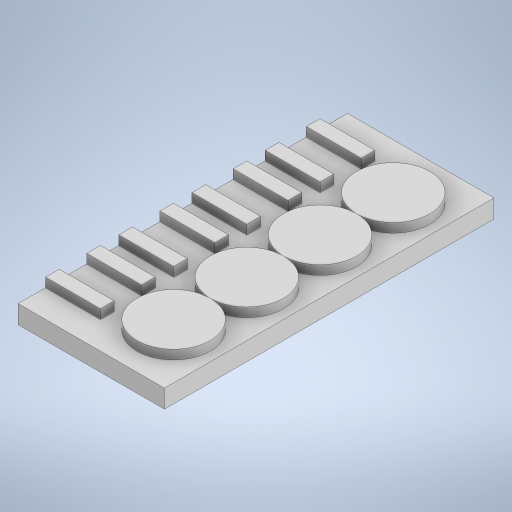
# Autodesk Inventor part: Zamysl na rekina
Saved by Autodesk Inventor 2024 (Build 280153000, 153)
## iProperties
Created: 2023-10-15
Part Number: Zamysl na rekina
Material: Generic
Document SubType Name: Modeling
Designer: Piter
Density: 1 g/cm^3
Appearance: Default
Author: Piter
Autodesk Inventor part; units mm, degrees
ref_plane "YZ Plane" through (0, 0, 0) normal (1, 0, 0) x (0, 1, 0)
ref_plane "XZ Plane" through (0, 0, 0) normal (0, 1, 0) x (-1, 0, 0)
ref_plane "XY Plane" through (0, 0, 0) normal (0, 0, 1) x (1, 0, 0)
sketch "Sketch1" plane through (0, 0, 0) normal (0, 1, 0) x (-1, 0, 0)
  line L0 (71.2912, 117.5402) -> (-8.7088, 117.5402)
  line L1 (-8.7088, 117.5402) -> (-8.7088, -62.4598)
  line L2 (-8.7088, -62.4598) -> (71.2912, -62.4598)
  line L3 (71.2912, -62.4598) -> (71.2912, 117.5402)
  point P0 (0, 0)
  dimension "d0" = 80
  dimension "d1" = 180
  constraints: 8 end point, 2 parallel, 1 horizontal, 1 perpendicular
  measures "d0" distance of L2.end L1.end
  measures "d1" distance of L1.end L0.end
extrude "Extrusion1" add sketch "Sketch1" along normal blind 10
sketch "Sketch2" plane through (0, 10, 0) normal (0, 1, 0) x (1, 0, 0)
  line L0 (8.7088, -117.5402) -> (8.7088, 62.4598) projected
  line L1 (8.7088, 62.4598) -> (-71.2912, 62.4598) projected
  line L2 (8.7088, -117.5402) -> (-16.2912, -117.5402)
  line L3 (-16.2912, 62.4598) -> (8.7088, 62.4598)
  line L4 (8.7088, 62.4598) -> (8.7088, -117.5402)
  line L5 (-16.2912, -117.5402) -> (-16.2912, -87.5402)
  circle A0 centre (-16.2912, -87.5402) radius 20
  circle A1 centre (-16.2912, -47.5402) radius 20
  circle A2 centre (-16.2912, -7.5402) radius 20
  circle A3 centre (-16.2912, 32.4598) radius 20
  line L6 (-16.2912, -87.5402) -> (-70.5888, -87.5402)
  line L7 (-71.2912, 62.4598) -> (-71.2912, -117.5402) projected
  line L8 (-41.2912, -95.0402) -> (-71.2912, -95.0402)
  line L9 (-71.2912, -95.0402) -> (-71.2912, -80.0402)
  line L10 (-71.2912, -80.0402) -> (-41.2912, -80.0402)
  line L11 (-41.2912, -80.0402) -> (-41.2912, -95.0402)
  line L12 (-41.2912, -95.0402) -> (-71.2912, -80.0402) construction
  line L13 (-71.2912, -95.0402) -> (-41.2912, -80.0402) construction
  line L14 (-71.2912, -95.0402) -> (-41.2912, -95.0402)
  line L15 (-41.2912, -95.0402) -> (-41.2912, -102.5402)
  line L16 (-41.2912, -102.5402) -> (-71.2912, -102.5402)
  line L17 (-71.2912, -102.5402) -> (-71.2912, -95.0402)
  line L18 (-71.2912, -80.0402) -> (-41.2912, -80.0402)
  line L19 (-41.2912, -80.0402) -> (-41.2912, -72.5402)
  line L20 (-41.2912, -72.5402) -> (-71.2912, -72.5402)
  line L21 (-71.2912, -72.5402) -> (-71.2912, -80.0402)
  line L22 (-41.2912, -40.0402) -> (-41.2912, -32.5402)
  line L23 (-41.2912, -32.5402) -> (-71.2912, -32.5402)
  line L24 (-71.2912, -32.5402) -> (-71.2912, -40.0402)
  line L25 (-71.2912, -40.0402) -> (-41.2912, -40.0402)
  line L26 (-71.2912, -40.0402) -> (-41.2912, -40.0402)
  line L27 (-41.2912, -40.0402) -> (-41.2912, -55.0402)
  line L28 (-41.2912, -55.0402) -> (-41.2912, -62.5402)
  line L29 (-71.2912, -55.0402) -> (-71.2912, -40.0402)
  line L30 (-71.2912, -55.0402) -> (-41.2912, -40.0402) construction
  line L31 (-71.2912, -55.0402) -> (-41.2912, -55.0402)
  line L32 (-41.2912, -55.0402) -> (-71.2912, -40.0402) construction
  line L33 (-71.2912, -62.5402) -> (-71.2912, -55.0402)
  line L34 (-41.2912, -62.5402) -> (-71.2912, -62.5402)
  line L35 (-41.2912, -0.0402) -> (-41.2912, 7.4598)
  line L36 (-41.2912, 7.4598) -> (-71.2912, 7.4598)
  line L37 (-71.2912, 7.4598) -> (-71.2912, -0.0402)
  line L38 (-71.2912, -0.0402) -> (-41.2912, -0.0402)
  line L39 (-71.2912, -0.0402) -> (-41.2912, -0.0402)
  line L40 (-41.2912, -0.0402) -> (-41.2912, -15.0402)
  line L41 (-41.2912, -15.0402) -> (-41.2912, -22.5402)
  line L42 (-71.2912, -15.0402) -> (-71.2912, -0.0402)
  line L43 (-71.2912, -15.0402) -> (-41.2912, -0.0402) construction
  line L44 (-71.2912, -15.0402) -> (-41.2912, -15.0402)
  line L45 (-41.2912, -15.0402) -> (-71.2912, -0.0402) construction
  line L46 (-71.2912, -22.5402) -> (-71.2912, -15.0402)
  line L47 (-41.2912, -22.5402) -> (-71.2912, -22.5402)
  line L48 (-41.2912, 39.9598) -> (-41.2912, 47.4598)
  line L49 (-41.2912, 47.4598) -> (-71.2912, 47.4598)
  line L50 (-71.2912, 47.4598) -> (-71.2912, 39.9598)
  line L51 (-71.2912, 39.9598) -> (-41.2912, 39.9598)
  line L52 (-71.2912, 39.9598) -> (-41.2912, 39.9598)
  line L53 (-41.2912, 39.9598) -> (-41.2912, 24.9598)
  line L54 (-41.2912, 24.9598) -> (-41.2912, 17.4598)
  line L55 (-71.2912, 24.9598) -> (-71.2912, 39.9598)
  line L56 (-71.2912, 24.9598) -> (-41.2912, 39.9598) construction
  line L57 (-71.2912, 24.9598) -> (-41.2912, 24.9598)
  line L58 (-41.2912, 24.9598) -> (-71.2912, 39.9598) construction
  line L59 (-71.2912, 17.4598) -> (-71.2912, 24.9598)
  line L60 (-41.2912, 17.4598) -> (-71.2912, 17.4598)
  point P0 (0, 0)
  point P1 (-16.2912, -27.5402)
  point P2 (-16.2912, 12.4598)
  point P3 (-16.2912, -27.5402)
  point P4 (-16.2912, -67.5402)
  point P5 (-56.2912, -87.5402)
  point P6 (-56.2912, -47.5402)
  point P7 (-70.5888, -47.5402)
  point P8 (-56.2912, -7.5402)
  point P9 (-70.5888, -7.5402)
  point P10 (-56.2912, 32.4598)
  point P11 (-70.5888, 32.4598)
  dimension "d4" = 25
  dimension "d5" = 30
  dimension "d6" = 40
  dimension "d7" = 40
  dimension "d8" = 40
  dimension "d9" = 40
  dimension "d10" = 40
  dimension "d12" = 40
  dimension "d13" = 40
  dimension "d14" = 25
  dimension "d17" = 15
  dimension "d18" = 30
  dimension "d19" = 7.5
  dimension "d22" = 40
  constraints: 116 end point, 36 vertical alignment, 28 parallel, 18 collinear, 6 point on line, 5 horizontal, 4 centre point, 3 perpendicular, 2 midpoint, 1 coincident, 2 other
  measures "d4" distance of L3.start L3.end
  measures "d5" distance of L2.end L5.end
  measures "d6" diameter of A0
  measures "d7" diameter of A1
  measures "d8" distance of A1.centre L5.end
  measures "d9" diameter of A2
  measures "d10" diameter of A3
  measures "d12" distance of A3.centre A2.centre
  measures "d13" distance of A1.centre A2.centre
  measures "d14" distance from line of L0 L5.end
  measures "d17" distance of L8.end L9.end
  measures "d18" distance of L9.end L10.end
  measures "d19" distance of L19.end L18.end
  measures "d22" distance of L19.end L22.end
extrude "Extrusion2" add sketch "Sketch2" along normal blind 5 contours A3 | A2 | A1 | A0 L6 L5 | L5 L6 A0 | L49 L48 L51 L7 | L10 L7 L20 L19 | L15 L16 L7 L8 | L57 L54 L60 L7 | L36 L35 L38 L7 | L7 L31 L28 L34 | L44 L41 L47 L7 | L7 L23 L22 L25
sketch "Sketch3" plane through (0, 10, 0) normal (0, 1, 0) x (1, 0, 0)
  point P0 (0, 0)
body "Solid1"
